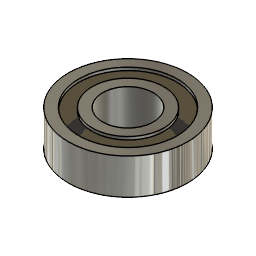
BoBRoss Assembly (Autodesk Fusion 360 archive; units mm, degrees)
design "bearing"
part number: 2026-08-11-22-14-24-283
Autodesk Fusion 360 part; units mm, degrees
sketch "Sketch2" plane through (0, 0, 0) normal (0, 0, 1) x (1, 0, 0)
  circle A0 centre (0, 0) radius 20
  circle A1 centre (0, 0) radius 8.5
  dimension "d1" = 40
  dimension "d2" = 17
  constraint coincident A0.centre A1.centre
  measures "d1" diameter of A0
  measures "d2" diameter of A1
extrude "Extrude1" add sketch "Sketch2" along normal blind 12
sketch "Sketch3" plane through (0, 0, 12) normal (0, 0, 1) x (-1, 0, 0)
  circle A0 centre (0, 0) radius 8.5
  circle A1 centre (0, 0) radius 20
  circle A2 centre (0, 0) radius 12
  circle A3 centre (0, 0) radius 16.5
  dimension "d5" = 24
  dimension "d6" = 33
  constraint coincident A0.centre A1.centre
  measures "d5" diameter of A2
  measures "d6" diameter of A3
extrude "Extrude2" cut sketch "Sketch3" against normal blind 1 contours A3
sketch "Sketch4" plane through (0, 0, 0) normal (0, 0, -1) x (1, 0, 0)
  circle A0 centre (0, 0) radius 8.5
  circle A1 centre (0, 0) radius 20
  circle A2 centre (0, 0) radius 12
  circle A3 centre (0, 0) radius 16.5
  dimension "d9" = 24
  dimension "d10" = 33
  constraint coincident A0.centre A1.centre
  measures "d9" diameter of A2
  measures "d10" diameter of A3
extrude "Extrude3" cut sketch "Sketch4" against normal blind 1 contours A3

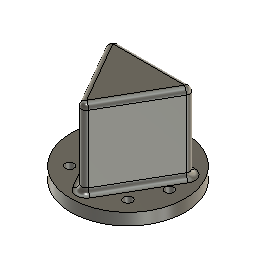
design "Servo_head_xm430"
part number: 2026-03-19-00-11-38-975
Autodesk Fusion 360 part; units mm, degrees
sketch "Sketch1" plane through (0, 0, 0) normal (0, 0, 1) x (1, 0, 0)
  circle A0 centre (0, 0) radius 11
  circle A1 centre (0, 8) radius 0.85
  circle A2 centre (-5.6569, 5.6569) radius 0.85
  circle A3 centre (-8, 0) radius 0.85
  circle A4 centre (-5.6569, -5.6569) radius 0.85
  circle A5 centre (0, -8) radius 0.85
  circle A6 centre (5.6569, -5.6569) radius 0.85
  circle A7 centre (8, 0) radius 0.85
  circle A8 centre (5.6569, 5.6569) radius 0.85
  circle A9 centre (0, 0) radius 4.25
  dimension "d1" = 22
  dimension "d2" = 1.7
  dimension "d3" = 8
  dimension "d5" = 360
  dimension "d6" = 8.5
  constraint coincident A0.centre A9.centre
  constraint concentric A0 A9
  measures "d1" diameter of A0
  measures "d2" diameter of A1
  measures "d3" distance of A0.centre A1.centre
  measures "d6" diameter of A9
extrude "Extrude1" add sketch "Sketch1" along normal blind 2.3 contours A0 | A2 | A5 | A8
sketch "Sketch8" plane through (0, 0, 2.3) normal (0, 0, 1) x (-1, 0, 0)
  circle A0 centre (0, 0) radius 4.25
  circle A1 centre (-5.6569, 5.6569) radius 0.85
  circle A2 centre (8, 0) radius 0.85
  circle A3 centre (5.6569, 5.6569) radius 0.85
  circle A4 centre (-8, 0) radius 0.85
  circle A5 centre (0, -8) radius 0.85
  circle A6 centre (0, 0) radius 11
  line L0 (0, 10) -> (-8.6603, -5)
  line L1 (-8.6603, -5) -> (8.6603, -5)
  line L2 (8.6603, -5) -> (0, 10)
  dimension "d52" = 60
  dimension "d53" = 60
  dimension "d54" = 5
  dimension "d55" = 5
  dimension "d56" = 5
  constraint horizontal L1
  measures "d52" angle of L0 L1
  measures "d53" angle of L1 L2
  measures "d54" distance of A0.centre L1
  measures "d55" distance of A0.centre L2
  measures "d56" distance of A0.centre L0
extrude "Extrude8" add sketch "Sketch8" along normal blind 15 contours A0 | L0 L1 L2
fillet "Fillet4" radius 1 3 edges at (8.6603, 5, 9.8) (-8.6603, 5, 9.8) (0, -10, 9.8)
fillet "Fillet4" radius 1 3 edges at (-4.3301, -2.5, 17.3) (4.3301, -2.5, 17.3) (0, 5, 17.3)
fillet "Fillet4" radius 1 3 edges at (-4.3301, -2.5, 2.3) (0, 5, 2.3) (4.3301, -2.5, 2.3)

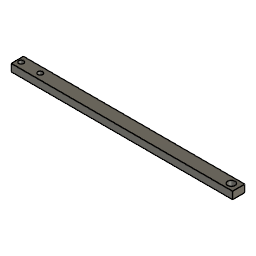
design "servo_stripper"
part number: 2026-09-03-23-44-18-717
Autodesk Fusion 360 part; units mm, degrees
sketch "Sketch1" plane through (0, 0, 0) normal (0, 0, 1) x (1, 0, 0)
  line L0 (0, 0) -> (90, 0)
  line L1 (90, 0) -> (90, 5)
  line L2 (90, 5) -> (0, 5)
  line L3 (0, 5) -> (0, 0)
  circle A0 centre (1.6, 2.5) radius 1
  circle A1 centre (9.333, 2.5) radius 1
  circle A2 centre (87, 2.5) radius 1.5
  dimension "d1" = 90
  dimension "d2" = 5
  dimension "d3" = 2
  dimension "d4" = 2
  dimension "d5" = 7.733
  dimension "d7" = 1.6
  dimension "d9" = 2.5
  dimension "d12" = 3
  dimension "d13" = 3
  constraint horizontal L0
  constraint vertical L1
  constraint horizontal L2
  constraint vertical L3
  constraint coincident L0.start L3.end
  constraint horizontal A0.centre A1.centre
  constraint horizontal A1.centre A2.centre
  measures "d1" distance of L0.start L0.end
  measures "d2" distance of L0.start L2.end
  measures "d3" diameter of A0
  measures "d4" diameter of A1
  measures "d5" horizontal distance of A0.centre A1.centre
  measures "d7" distance of L3 A0.centre
  measures "d9" vertical distance of L0.start A0.centre
  measures "d12" diameter of A2
  measures "d13" distance of L1 A2.centre
extrude "Extrude1" add sketch "Sketch1" along normal blind 3

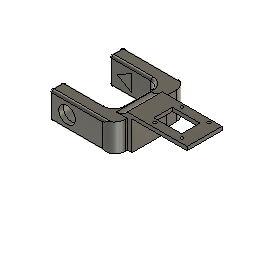
design "link3"
part number: 2026-08-23-14-44-17-445
Autodesk Fusion 360 part; units mm, degrees
sketch "Sketch1" plane through (0, 0, 0) normal (0, 0, 1) x (1, 0, 0)
  line L0 (0, 0) -> (5, 0)
  line L1 (5, 0) -> (5, 25)
  line L2 (5, 25) -> (0, 25)
  line L3 (0, 25) -> (0, 0)
  line L4 (-15, 52.5) -> (0, 52.5)
  line L5 (0, 52.5) -> (0, -27.5)
  line L6 (0, -27.5) -> (-15, -27.5)
  line L7 (-15, -27.5) -> (-15, 52.5)
  line L8 (-15, 52.5) -> (-70, 52.5)
  line L9 (-70, 52.5) -> (-70, 37.5)
  line L10 (-70, 37.5) -> (-15, 37.5)
  line L11 (-15, 37.5) -> (-15, 52.5)
  line L12 (-15, -27.5) -> (-70, -27.5)
  line L13 (-70, -27.5) -> (-70, -12.5)
  line L14 (-70, -12.5) -> (-15, -12.5)
  line L15 (-15, -12.5) -> (-15, -27.5)
  dimension "d1" = 25
  dimension "d2" = 15
  dimension "d3" = 15
  dimension "d4" = 80
  dimension "d6" = 27.5
  dimension "d7" = 15
  dimension "d8" = 15
  dimension "d9" = 5
  dimension "d14" = 55
  dimension "d15" = 55
  constraint horizontal L0
  constraint vertical L1
  constraint horizontal L2
  constraint vertical L3
  constraint coincident L0.start L3.end
  constraint horizontal L4
  constraint vertical L5
  constraint horizontal L6
  constraint vertical L7
  constraint horizontal L8
  constraint vertical L9
  constraint horizontal L10
  constraint vertical L11
  constraint horizontal L12
  constraint vertical L13
  constraint horizontal L14
  constraint vertical L15
  measures "d1" distance of L0.start L2.end
  measures "d2" distance of L4.start L4.end
  measures "d3" distance of L3 L7
  measures "d4" distance of L4.start L6.end
  measures "d6" distance of L2 L4
  measures "d7" distance of L8.end L9.end
  measures "d8" distance of L12.end L13.end
  measures "d9" distance of L1.end L2.end
  measures "d14" distance of L13.end L14.end
  measures "d15" distance of L9.end L10.end
extrude "Extrude1" add sketch "Sketch1" along normal blind 30 makes body 1
sketch "Sketch2" plane through (0, -12.5, 0) normal (0, 1, 0) x (-1, 0, 0)
  line L0 (15, 0) -> (70, 0)
  line L1 (70, 0) -> (70, 30)
  line L2 (70, 30) -> (15, 30)
  line L3 (15, 30) -> (15, 0)
  circle A0 centre (51, 15) radius 12.1
  circle A1 centre (51, 15) radius 9
  dimension "d12" = 24.2
  dimension "d13" = 36
  dimension "d16" = 18
  constraint concentric A0 A1
  measures "d12" diameter of A0
  measures "d13" distance of L3 A0.centre
  measures "d16" diameter of A1
extrude "Extrude2" cut sketch "Sketch2" against normal blind 15 contours A1 bodies 1
extrude "Extrude3" cut sketch "Sketch2" against normal blind 10 contours A0 bodies 1
sketch "Sketch3" plane through (0, 37.5, 0) normal (0, -1, 0) x (1, 0, 0)
  line L0 (-70, 0) -> (-15, 0)
  line L1 (-15, 0) -> (-15, 30)
  line L2 (-15, 30) -> (-70, 30)
  line L3 (-70, 30) -> (-70, 0)
  line L4 (-45.8, 24.0067) -> (-61.4, 15)
  line L5 (-61.4, 15) -> (-45.8, 5.9933)
  line L6 (-45.8, 5.9933) -> (-45.8, 24.0067)
  point P0 (-51, 15)
  dimension "d21" = 5.2
  dimension "d22" = 36
  dimension "d23" = 360
  dimension "d26" = 15
  measures "d21" distance of P0 L6
  measures "d22" distance of L1 P0
  measures "d26" distance of L0 P0
extrude "Extrude4" cut sketch "Sketch3" against normal blind 15 contours L4 L5 L6 bodies 1
fillet "Fillet1" radius 10 2 edges at (-15, 37.5, 15) (-15, -12.5, 15) on bodies 1
fillet "Fillet1" radius 12.5 2 edges at (0, -27.5, 15) (0, 52.5, 15) on bodies 1
fillet "Fillet1" radius 2.5 4 edges at (-70, -27.5, 15) (-70, -12.5, 15) (-70, 37.5, 15) (-70, 52.5, 15) on bodies 1
fillet "Fillet1" radius 2.5 7 edges at (-42.5, -12.5, 0) (-35, -27.5, 0) (-15, 12.5, 0) (-42.5, 37.5, 0) (-35, 52.5, 0) (-70, 45, 0) (-70, -20, 0) on bodies 1
fillet "Fillet1" radius 2.5 7 edges at (-42.5, 37.5, 30) (-70, 45, 30) (-35, 52.5, 30) (-15, 12.5, 30) (-42.5, -12.5, 30) (-70, -20, 30) (-35, -27.5, 30) on bodies 1
sketch "Sketch8" plane through (5, 0, 0) normal (1, 0, 0) x (0, 1, 0)
  line L0 (0, 0) -> (25, 0)
  line L1 (25, 0) -> (25, 30)
  line L2 (25, 30) -> (0, 30)
  line L3 (0, 30) -> (0, 0)
  line L4 (-13, 31.9) -> (25, 31.9)
  line L5 (25, 31.9) -> (25, 35.9)
  line L6 (25, 35.9) -> (-13, 35.9)
  line L7 (-13, 35.9) -> (-13, 31.9)
  line L8 (22.0304, 15) -> (-72.0304, 15)
  line L9 (25, 31.9) -> (25, 31.9)
  line L10 (25, 30) -> (25, 30)
  line L11 (25, 30) -> (25, 31.9)
  line L12 (-13, 31.9) -> (-13, 30)
  line L13 (-13, 30) -> (0, 30)
  dimension "d85" = 16.9
  dimension "d86" = 38
  dimension "d87" = 4
  constraint horizontal L4
  constraint vertical L5
  constraint horizontal L6
  constraint vertical L7
  constraint coincident L1.end L2.start
  constraint perpendicular L4 L12
  constraint coincident L2.end L3.start
  constraint perpendicular L3 L13
  measures "d85" distance of L4 L8
  measures "d86" distance of L5.end L6.end
  measures "d87" distance of L4.start L6.end
extrude "Extrude9" add sketch "Sketch8" against normal blind 5 separate body contours L2 L4 L11 L12 L13 makes body 2
extrude "Extrude10" add sketch "Sketch8" along normal blind 60 separate body contours L4 L5 L6 L7 makes body 3
extrude "Extrude11" add sketch "Sketch8" against normal blind 5 contours L4 L5 L6 L7 bodies 2 3
sketch "Sketch9" plane through (0, 0, 31.9) normal (0, 0, -1) x (1, 0, 0)
  line L0 (5, 13) -> (5, -25)
  line L1 (5, -25) -> (65, -25)
  line L2 (65, -25) -> (65, 13)
  line L3 (65, 13) -> (5, 13)
  line L4 (50, -16) -> (20, -16)
  line L5 (20, -16) -> (20, 4)
  line L6 (20, 4) -> (50, 4)
  line L7 (50, 4) -> (50, -16)
  circle A0 centre (25, -21.5) radius 1.6
  circle A1 centre (25, 7.9) radius 1.6
  circle A2 centre (54.3, -21.5) radius 1.6
  circle A3 centre (54.3, 7.9) radius 1.6
  line L8 (5, 13) -> (5, -25)
  line L9 (5, 13) -> (5, 0)
  dimension "d94" = 3.2
  dimension "d95" = 3.2
  dimension "d96" = 3.2
  dimension "d97" = 3.2
  dimension "d98" = 20
  dimension "d99" = 9
  dimension "d100" = 29.4
  dimension "d101" = 3.5
  dimension "d102" = 29.4
  dimension "d103" = 3.5
  dimension "d104" = 20
  dimension "d105" = 29.3
  dimension "d106" = 20
  dimension "d107" = 29.3
  dimension "d108" = 15
  dimension "d109" = 30
  constraint horizontal L4
  constraint vertical L5
  constraint horizontal L6
  constraint vertical L7
  measures "d94" diameter of A2
  measures "d95" diameter of A0
  measures "d96" diameter of A3
  measures "d97" diameter of A1
  measures "d98" distance of L4.start L6.end
  measures "d99" distance of L1 L4
  measures "d100" distance of A0.centre A1.centre
  measures "d101" distance of L1 A0.centre
  measures "d102" distance of A2.centre A3.centre
  measures "d103" distance of L1 A2.centre
  measures "d104" distance of A0.centre L8
  measures "d105" distance of A0.centre A2.centre
  measures "d106" distance of A1.centre L9
  measures "d107" distance of A1.centre A3.centre
  measures "d108" distance of L5 L8
  measures "d109" distance of L4.start L4.end
extrude "Extrude12" cut sketch "Sketch9" against normal blind 4 contours L4 L5 L6 L7 | A0 | A1 | A2 | A3 bodies 2
extrude "Extrude13" add 1 faces at (1.6667, 0, 10) along direction (0, -1, 0) blind 13 on bodies 1 bodies 1 2
fillet "Fillet6" radius 15 1 edges at (0, 6, 30) on bodies 1
equation "d100 = 22.4 mm + 7 mm"
equation "d105 = 42.3 mm - 13 mm"
